Guitar grommet (Autodesk Fusion 360 design; units mm, degrees)
Autodesk Fusion 360 part; units mm, degrees
sketch "Sketch1" plane through (0, 0, 0) normal (0, 1, 0) x (1, 0, 0)
  line L0 (0, -10) -> (0, 10)
  line L1 (2, -3.729) -> (2, 4.421)
  line L2 (2, 4.421) -> (3.5, 4.421)
  line L3 (3.85, -5.579) -> (6.0767, -5.579)
  line L4 (3.5, 4.421) -> (3.5, -5.229)
  line L5 (7.5, -4.3954) -> (7.5, -3.7633)
  line L6 (5.4261, -2.579) -> (3.5, -2.579)
  line L7 (3.5, 4.421) -> (5, 4.421)
  line L8 (5, 4.421) -> (5, 1.921)
  line L9 (5, 1.921) -> (3.3307, 1.921)
  arc A0 (6.0767, -5.579) -> (7.1665, -3.096) centre (6.0334, -4.0794) ccw
  spline S0 degree 5 poles (7.1665, -3.096) (6.933, -3.0417) (6.4824, -2.9292) (5.8552, -2.7485) (5.1184, -2.4835) (4.3745, -2.1094) (3.9119, -1.7552) (3.6679, -1.4589) (3.5538, -1.242) (3.5075, -1.1195) (3.5, -1.0984) knots 0 0 0 0 0 0 0.1 0.2 0.3 0.4 0.5 0.520654 0.520654 0.520654 0.520654 0.520654 0.520654
  line L10 (3.5931, -1.3616) -> (3.4069, -0.8351)
  spline S1 degree 5 poles (3.5, -0.1837) (3.505, -0.1666) (3.547, -0.0298) (3.6508, 0.2328) (3.8703, 0.6342) (4.183, 1.0582) (4.561, 1.4822) (4.8479, 1.7733) (5, 1.921) knots 0.685718 0.685718 0.685718 0.685718 0.685718 0.685718 0.7 0.8 0.9 1 1 1 1 1 1
  line L11 (3.4418, -0.381) -> (3.5582, 0.0137)
  line L12 (3.85, -5.579) -> (9.2988, -5.579) construction
  line L13 (3.85, -5.579) -> (2, -3.729)
  line L14 (0, -1.729) -> (-0.0029, -1.7262)
  dimension "d1" = 2
  dimension "d3" = 1.5
  dimension "d6" = 1.5
  dimension "d7" = 2.5
  dimension "d9" = 135
  constraint vertical L0
  constraint vertical L1
  constraint perpendicular L1 L2
  constraint perpendicular L1 L3
  constraint perpendicular L3 L4
  constraint perpendicular L3 L5
  constraint coincident L4 L6.end
  constraint perpendicular L4 L6
  constraint perpendicular L4 L7
  constraint perpendicular L7 L8
  constraint perpendicular L8 L9
  constraint tangent L6 A0
  constraint coincident A0 L5.start
  constraint coincident A0 L5.end
  constraint coincident L6.start S0
  constraint coincident L4 S0.end
  constraint midpoint S0.end L10
  constraint coincident L4 S1.start
  constraint midpoint S1.start L11
  constraint horizontal L12
  constraint coincident L0 L14.start
  constraint collinear L13 L14
  constraint coincident L13 L4.end
  measures "d1" distance of L0 L1
  measures "d3" distance of L1.end L2.end
  measures "d6" distance of L2.end L7.end
  measures "d7" distance of L7.end L8.end
  measures "d9" angle of L12 L13
revolve "Revolve1" add sketch "Sketch1" angle 360 about axis through (0, 0, 10) along (0, 0, -1) contours L1 L2 L4 L13 | L3 L4 L5 L6 A0 S0 L13 | L4 L7 L8 L9 | L4 L6 S0 | L4 L9 S1
